Autodesk Fusion 360 part; units mm, degrees
(part 4 of 7)
  spline S1051 degree 3 poles (80.1455, 58.4684) (80.4873, 58.6658) (80.7712, 58.9498) (80.9687, 59.2916) knots 0 0 0 0 1 1 1 1
  spline S1052 degree 3 poles (81.2136, 60.9174) (81.1761, 61.0816) (81.1203, 61.241) (81.0472, 61.3928) knots 0 0 0 0 1 1 1 1
  spline S1053 degree 3 poles (81.2705, 60.4166) (81.2703, 60.5851) (81.2513, 60.7531) (81.2136, 60.9174) knots 0 0 0 0 1 1 1 1
  line L303 (70.73, 56.4437) -> (69.42, 56.4437)
  spline S1054 degree 3 poles (81.0472, 61.3928) (80.9743, 61.5446) (80.8845, 61.6878) (80.7795, 61.8196) knots 0 0 0 0 1 1 1 1
  spline S1055 degree 3 poles (80.7795, 61.8196) (80.6744, 61.9513) (80.5548, 62.0707) (80.423, 62.1757) knots 0 0 0 0 1 1 1 1
  spline S1056 degree 3 poles (79.9966, 62.4439) (79.8447, 62.517) (79.6851, 62.5728) (79.5207, 62.6103) knots 0 0 0 0 1 1 1 1
  line L304 (75.5752, 64.5037) -> (75.5752, 64.5037)
  spline S1057 degree 3 poles (68.6407, 56.8938) (68.8015, 56.6154) (69.0985, 56.4438) (69.42, 56.4437) knots 0 0 0 0 1 1 1 1
  spline S1058 degree 3 poles (71.5093, 57.7935) (71.3486, 58.072) (71.0515, 58.2436) (70.73, 58.2436) knots 0 0 0 0 1 1 1 1
  spline S1059 degree 3 poles (68.0149, 63.2438) (68.015, 62.6974) (68.2321, 62.1734) (68.6185, 61.7871) knots 0 0 0 0 1 1 1 1
  line L305 (79.0205, 62.6666) -> (79.0205, 62.6666)
  spline S1060 degree 3 poles (70.0753, 61.1835) (70.2552, 61.1836) (70.4343, 61.2072) (70.6081, 61.2538) knots 0 0 0 0 1 1 1 1
  spline S1061 degree 3 poles (71.1052, 61.4594) (71.261, 61.5496) (71.4043, 61.6597) (71.5315, 61.7871) knots 0 0 0 0 1 1 1 1
  spline S1062 degree 3 poles (71.1052, 65.0277) (70.9492, 65.1177) (70.7821, 65.1868) (70.6081, 65.2334) knots 0 0 0 0 1 1 1 1
  spline S1063 degree 3 poles (71.8592, 64.2737) (71.769, 64.4296) (71.6589, 64.5729) (71.5315, 64.7001) knots 0 0 0 0 1 1 1 1
  spline S1064 degree 3 poles (80.423, 62.1757) (80.2913, 62.2808) (80.1483, 62.3707) (79.9966, 62.4439) knots 0 0 0 0 1 1 1 1
  spline S1065 degree 3 poles (79.5207, 62.6103) (79.6851, 62.5728) (79.8447, 62.517) (79.9966, 62.4439) knots 0 0 0 0 1 1 1 1
  spline S1066 degree 3 poles (74.6843, 62.3524) (74.9206, 62.1162) (75.2411, 61.9834) (75.5752, 61.9834) knots 0 0 0 0 1 1 1 1
  spline S1067 degree 3 poles (77.0718, 59.2916) (77.2693, 58.9497) (77.5534, 58.6658) (77.8955, 58.4684) knots 0 0 0 0 1 1 1 1
  spline S1068 degree 3 poles (79.5207, 62.6103) (79.3566, 62.6477) (79.1888, 62.6666) (79.0205, 62.6666) knots 0 0 0 0 1 1 1 1
  line L306 (69.42, 56.4437) -> (70.73, 56.4437)
  line L307 (70.73, 58.2436) -> (69.42, 58.2436)
  spline S1069 degree 3 poles (68.6407, 57.7935) (68.8015, 58.072) (69.0985, 58.2436) (69.42, 58.2436) knots 0 0 0 0 1 1 1 1
  spline S1070 degree 3 poles (70.73, 58.2436) (71.0515, 58.2436) (71.3486, 58.072) (71.5093, 57.7935) knots 0 0 0 0 1 1 1 1
  spline S1071 degree 3 poles (70.0753, 65.3037) (69.5289, 65.3036) (69.0048, 65.0865) (68.6185, 64.7001) knots 0 0 0 0 1 1 1 1
  spline S1072 degree 3 poles (68.6185, 64.7001) (68.2322, 64.3139) (68.0151, 63.7901) (68.0149, 63.2438) knots 0 0 0 0 1 1 1 1
  spline S1073 degree 3 poles (70.6081, 61.2538) (70.7821, 61.3003) (70.9492, 61.3695) (71.1052, 61.4594) knots 0 0 0 0 1 1 1 1
  spline S1074 degree 3 poles (74.3148, 63.2438) (74.3148, 62.9094) (74.4477, 62.5887) (74.6843, 62.3524) knots 0 0 0 0 1 1 1 1
  spline S1075 degree 3 poles (76.7736, 63.633) (76.7326, 63.7588) (76.6721, 63.8774) (76.5943, 63.9844) knots 0 0 0 0 1 1 1 1
  line L308 (69.42, 58.2436) -> (70.73, 58.2436)
  spline S1076 degree 3 poles (72.0648, 63.7766) (72.0183, 63.9506) (71.9492, 64.1177) (71.8592, 64.2737) knots 0 0 0 0 1 1 1 1
  spline S1077 degree 3 poles (71.5315, 61.7871) (71.6589, 61.9143) (71.769, 62.0576) (71.8592, 62.2134) knots 0 0 0 0 1 1 1 1
  spline S1078 degree 3 poles (71.8592, 62.2134) (71.9492, 62.3694) (72.0183, 62.5365) (72.0648, 62.7105) knots 0 0 0 0 1 1 1 1
  line L309 (70.0753, 65.3037) -> (70.0753, 65.3037)
  spline S1079 degree 3 poles (76.8351, 63.2438) (76.8351, 63.376) (76.8144, 63.5073) (76.7736, 63.633) knots 0 0 0 0 1 1 1 1
  spline S1080 degree 3 poles (74.6843, 64.1347) (74.4479, 63.8985) (74.3149, 63.578) (74.3148, 63.2438) knots 0 0 0 0 1 1 1 1
  spline S1081 degree 3 poles (75.9643, 64.4417) (75.8387, 64.4826) (75.7074, 64.5036) (75.5752, 64.5037) knots 0 0 0 0 1 1 1 1
  spline S1082 degree 3 poles (70.73, 56.4437) (71.0515, 56.4438) (71.3486, 56.6154) (71.5093, 56.8938) knots 0 0 0 0 1 1 1 1
  spline S1083 degree 3 poles (68.6185, 61.7871) (69.0048, 61.4006) (69.5289, 61.1835) (70.0753, 61.1835) knots 0 0 0 0 1 1 1 1
  spline S1084 degree 3 poles (47.4048, 61.1856) (47.4049, 60.6391) (47.622, 60.1151) (48.0084, 59.7288) knots 0 0 0 0 1 1 1 1
  spline S1085 degree 3 poles (48.0084, 59.7288) (48.3946, 59.3425) (48.9184, 59.1254) (49.4647, 59.1252) knots 0 0 0 0 1 1 1 1
  spline S1086 degree 3 poles (46.1264, 56.7548) (45.9805, 56.4683) (45.6929, 56.2814) (45.3719, 56.2644) knots 0 0 0 0 1 1 1 1
  line L310 (49.1665, 54.3607) -> (50.4749, 54.4289)
  spline S1087 degree 3 poles (49.4647, 63.2454) (48.9185, 63.2454) (48.3947, 63.0284) (48.0084, 62.6423) knots 0 0 0 0 1 1 1 1
  spline S1088 degree 3 poles (49.4647, 59.1252) (49.6447, 59.1252) (49.824, 59.1489) (49.998, 59.1955) knots 0 0 0 0 1 1 1 1
  spline S1089 degree 3 poles (49.0724, 56.158) (48.752, 56.1404) (48.4651, 55.9536) (48.3195, 55.6676) knots 0 0 0 0 1 1 1 1
  spline S1090 degree 3 poles (51.2491, 60.1557) (51.339, 60.3115) (51.4081, 60.4785) (51.4547, 60.6523) knots 0 0 0 0 1 1 1 1
  line L311 (50.4749, 54.4289) -> (49.1665, 54.3607)
  spline S1091 degree 3 poles (51.4547, 60.6523) (51.5014, 60.8262) (51.525, 61.0055) (51.525, 61.1856) knots 0 0 0 0 1 1 1 1
  spline S1092 degree 3 poles (48.3665, 54.7699) (48.5411, 54.5006) (48.8459, 54.3447) (49.1665, 54.3607) knots 0 0 0 0 1 1 1 1
  spline S1093 degree 3 poles (79.9966, 62.4439) (80.1483, 62.3707) (80.2913, 62.2808) (80.423, 62.1757) knots 0 0 0 0 1 1 1 1
  spline S1094 degree 3 poles (50.4749, 54.4289) (50.7957, 54.4463) (51.0828, 54.6334) (51.2284, 54.9198) knots 0 0 0 0 1 1 1 1
  line L312 (50.3804, 56.2267) -> (50.3804, 56.2267)
  spline S1095 degree 3 poles (50.9214, 59.7288) (51.0488, 59.8561) (51.159, 59.9997) (51.2491, 60.1557) knots 0 0 0 0 1 1 1 1
  spline S1096 degree 3 poles (51.4547, 61.7189) (51.4081, 61.8927) (51.339, 62.0596) (51.2491, 62.2155) knots 0 0 0 0 1 1 1 1
  spline S1097 degree 3 poles (79.0205, 62.6666) (79.1888, 62.6666) (79.3566, 62.6477) (79.5207, 62.6103) knots 0 0 0 0 1 1 1 1
  spline S1098 degree 3 poles (50.9214, 62.6423) (50.7942, 62.7695) (50.6509, 62.8795) (50.4951, 62.9694) knots 0 0 0 0 1 1 1 1
  spline S1099 degree 3 poles (80.1455, 58.4684) (79.8035, 58.2708) (79.4155, 58.1667) (79.0205, 58.1666) knots 0 0 0 0 1 1 1 1
  spline S1100 degree 3 poles (46.0793, 57.6535) (46.2544, 57.3838) (46.2723, 57.0413) (46.1264, 56.7548) knots 0 0 0 0 1 1 1 1
  spline S1101 degree 3 poles (46.0793, 57.6535) (45.9042, 57.9232) (45.5985, 58.0791) (45.2773, 58.0622) knots 0 0 0 0 1 1 1 1
  spline S1102 degree 3 poles (54.0664, 62.3643) (53.8302, 62.128) (53.6975, 61.8075) (53.6975, 61.4734) knots 0 0 0 0 1 1 1 1
  spline S1103 degree 3 poles (51.2284, 54.9198) (51.0828, 54.6334) (50.7957, 54.4463) (50.4749, 54.4289) knots 0 0 0 0 1 1 1 1
  spline S1104 degree 3 poles (53.6975, 61.4734) (53.6975, 61.1393) (53.8302, 60.8188) (54.0664, 60.5825) knots 0 0 0 0 1 1 1 1
  line L313 (43.9694, 57.9935) -> (45.2773, 58.0622)
  spline S1105 degree 3 poles (49.998, 59.1955) (50.172, 59.2422) (50.3391, 59.3115) (50.4951, 59.4017) knots 0 0 0 0 1 1 1 1
  spline S1106 degree 3 poles (54.9574, 62.7333) (54.6232, 62.7333) (54.3027, 62.6006) (54.0664, 62.3643) knots 0 0 0 0 1 1 1 1
  spline S1107 degree 3 poles (51.2491, 62.2155) (51.159, 62.3715) (51.0488, 62.515) (50.9214, 62.6423) knots 0 0 0 0 1 1 1 1
  line L314 (50.3804, 56.2267) -> (49.0724, 56.158)
  spline S1108 degree 3 poles (50.4951, 62.9694) (50.3391, 63.0594) (50.172, 63.1286) (49.998, 63.1751) knots 0 0 0 0 1 1 1 1
  spline S1109 degree 3 poles (51.525, 61.1856) (51.525, 61.3656) (51.5014, 61.5449) (51.4547, 61.7189) knots 0 0 0 0 1 1 1 1
  spline S1110 degree 3 poles (54.9574, 60.2135) (55.2915, 60.2135) (55.612, 60.3462) (55.8483, 60.5825) knots 0 0 0 0 1 1 1 1
  spline S1111 degree 3 poles (80.423, 62.1757) (80.5548, 62.0707) (80.6744, 61.9513) (80.7795, 61.8196) knots 0 0 0 0 1 1 1 1
  line L315 (45.3719, 56.2644) -> (44.0634, 56.1957)
  spline S1112 degree 3 poles (80.9687, 59.2916) (80.7712, 58.9498) (80.4873, 58.6658) (80.1455, 58.4684) knots 0 0 0 0 1 1 1 1
  spline S1113 degree 3 poles (50.4951, 59.4017) (50.6509, 59.4916) (50.7942, 59.6016) (50.9214, 59.7288) knots 0 0 0 0 1 1 1 1
  spline S1114 degree 3 poles (51.1814, 55.8174) (51.0066, 56.087) (50.7013, 56.243) (50.3804, 56.2267) knots 0 0 0 0 1 1 1 1
  spline S1115 degree 3 poles (50.3804, 56.2267) (50.7013, 56.243) (51.0066, 56.087) (51.1814, 55.8174) knots 0 0 0 0 1 1 1 1
  spline S1116 degree 3 poles (49.998, 63.1751) (49.824, 63.2217) (49.6447, 63.2454) (49.4647, 63.2454) knots 0 0 0 0 1 1 1 1
  spline S1117 degree 3 poles (54.0664, 60.5825) (54.3027, 60.3462) (54.6232, 60.2135) (54.9574, 60.2135) knots 0 0 0 0 1 1 1 1
  spline S1118 degree 3 poles (56.2172, 61.4734) (56.2173, 61.6055) (56.1965, 61.7368) (56.1557, 61.8625) knots 0 0 0 0 1 1 1 1
  spline S1119 degree 3 poles (56.1557, 61.8625) (56.1149, 61.9883) (56.0546, 62.1069) (55.9769, 62.2139) knots 0 0 0 0 1 1 1 1
  spline S1120 degree 3 poles (48.3195, 55.6676) (48.174, 55.3814) (48.1919, 55.0393) (48.3665, 54.7699) knots 0 0 0 0 1 1 1 1
  spline S1121 degree 3 poles (48.3665, 54.7699) (48.1919, 55.0393) (48.174, 55.3814) (48.3195, 55.6676) knots 0 0 0 0 1 1 1 1
  spline S1122 degree 3 poles (55.8483, 60.5825) (56.0845, 60.8188) (56.2172, 61.1393) (56.2172, 61.4734) knots 0 0 0 0 1 1 1 1
  spline S1123 degree 3 poles (81.0472, 61.3928) (81.1203, 61.241) (81.1761, 61.0816) (81.2136, 60.9174) knots 0 0 0 0 1 1 1 1
  spline S1124 degree 3 poles (45.2773, 58.0622) (45.5985, 58.0791) (45.9042, 57.9232) (46.0793, 57.6535) knots 0 0 0 0 1 1 1 1
  spline S1125 degree 3 poles (44.0634, 56.1957) (43.7427, 56.1795) (43.4377, 56.3355) (43.263, 56.605) knots 0 0 0 0 1 1 1 1
  spline S1126 degree 3 poles (51.2284, 54.9198) (51.3739, 55.206) (51.356, 55.548) (51.1814, 55.8174) knots 0 0 0 0 1 1 1 1
  spline S1127 degree 3 poles (48.0084, 62.6423) (47.622, 62.256) (47.4049, 61.732) (47.4048, 61.1856) knots 0 0 0 0 1 1 1 1
  spline S1128 degree 3 poles (55.9769, 62.2139) (55.8991, 62.3208) (55.8049, 62.4148) (55.6979, 62.4925) knots 0 0 0 0 1 1 1 1
  spline S1129 degree 3 poles (81.2136, 60.9174) (81.2513, 60.7531) (81.2703, 60.5851) (81.2705, 60.4166) knots 0 0 0 0 1 1 1 1
  spline S1130 degree 3 poles (48.3195, 55.6676) (48.4651, 55.9536) (48.752, 56.1404) (49.0724, 56.158) knots 0 0 0 0 1 1 1 1
  line L316 (49.4647, 63.2454) -> (49.4647, 63.2454)
  spline S1131 degree 3 poles (55.6979, 62.4925) (55.5909, 62.5703) (55.4723, 62.6308) (55.3465, 62.6718) knots 0 0 0 0 1 1 1 1
  spline S1132 degree 3 poles (83.1639, 74.4375) (82.8425, 74.4431) (82.5425, 74.2768) (82.3769, 74.0013) knots 0 0 0 0 1 1 1 1
  spline S1133 degree 3 poles (81.2705, 60.4166) (81.2704, 60.0216) (81.1663, 59.6336) (80.9687, 59.2916) knots 0 0 0 0 1 1 1 1
  spline S1134 degree 3 poles (49.1665, 54.3607) (48.8459, 54.3447) (48.5411, 54.5006) (48.3665, 54.7699) knots 0 0 0 0 1 1 1 1
  spline S1135 degree 3 poles (80.7795, 61.8196) (80.8845, 61.6878) (80.9743, 61.5446) (81.0472, 61.3928) knots 0 0 0 0 1 1 1 1
  spline S1136 degree 3 poles (51.1814, 55.8174) (51.356, 55.548) (51.3739, 55.206) (51.2284, 54.9198) knots 0 0 0 0 1 1 1 1
  line L317 (45.2773, 58.0622) -> (45.2773, 58.0622)
  spline S1137 degree 3 poles (43.216, 57.5031) (43.3616, 57.7893) (43.6487, 57.9762) (43.9694, 57.9935) knots 0 0 0 0 1 1 1 1
  spline S1138 degree 3 poles (43.263, 56.605) (43.0881, 56.8745) (43.0702, 57.2168) (43.216, 57.5031) knots 0 0 0 0 1 1 1 1
  line L318 (49.0724, 56.158) -> (50.3804, 56.2267)
  line L319 (64.4203, 60.3438) -> (65.7303, 60.3438)
  spline S1139 degree 3 poles (65.7303, 60.3438) (66.0518, 60.3437) (66.3489, 60.1721) (66.5096, 59.8937) knots 0 0 0 0 1 1 1 1
  spline S1140 degree 3 poles (66.5096, 58.9934) (66.6705, 59.272) (66.6705, 59.6151) (66.5096, 59.8937) knots 0 0 0 0 1 1 1 1
  line L320 (64.4203, 58.5439) -> (65.7303, 58.5439)
  spline S1141 degree 3 poles (65.4663, 62.3524) (65.7026, 62.5888) (65.8354, 62.9095) (65.8352, 63.2438) knots 0 0 0 0 1 1 1 1
  spline S1142 degree 3 poles (64.4203, 58.5439) (64.0987, 58.5436) (63.8015, 58.715) (63.6405, 58.9934) knots 0 0 0 0 1 1 1 1
  spline S1143 degree 3 poles (65.8352, 63.2438) (65.8351, 63.376) (65.8142, 63.5073) (65.7732, 63.633) knots 0 0 0 0 1 1 1 1
  spline S1144 degree 3 poles (43.1705, 60.4166) (43.1703, 60.2725) (43.1563, 60.1287) (43.1286, 59.9872) knots 0 0 0 0 1 1 1 1
  line L321 (67.0651, 54.4439) -> (67.0651, 54.9234)
  spline S1145 degree 3 poles (64.5748, 64.5037) (64.2407, 64.5037) (63.9202, 64.371) (63.6839, 64.1347) knots 0 0 0 0 1 1 1 1
  line L322 (70.0851, 48.9434) -> (68.4852, 48.9434)
  spline S1146 degree 3 poles (85.2273, 73.052) (85.3924, 73.3274) (85.3983, 73.6698) (85.2428, 73.9507) knots 0 0 0 0 1 1 1 1
  spline S1147 degree 3 poles (85.2428, 73.9507) (85.0874, 74.2315) (84.7943, 74.4083) (84.4734, 74.4147) knots 0 0 0 0 1 1 1 1
  spline S1148 degree 3 poles (65.7732, 63.633) (65.7324, 63.7587) (65.6721, 63.8773) (65.5944, 63.9844) knots 0 0 0 0 1 1 1 1
  spline S1149 degree 3 poles (63.6405, 58.9934) (63.4797, 59.272) (63.4797, 59.6151) (63.6405, 59.8937) knots 0 0 0 0 1 1 1 1
  line L323 (68.4852, 48.9434) -> (67.5349, 49.8436)
  spline S1150 degree 3 poles (112.8644, 55.9265) (112.9902, 55.8855) (113.1088, 55.825) (113.2158, 55.7471) knots 0 0 0 0 1 1 1 1
  line L324 (65.7303, 58.5439) -> (64.4203, 58.5439)
  spline S1151 degree 3 poles (43.1136, 60.9174) (43.1513, 60.7531) (43.1703, 60.5851) (43.1705, 60.4166) knots 0 0 0 0 1 1 1 1
  spline S1152 degree 3 poles (63.6405, 58.9934) (63.8015, 58.715) (64.0987, 58.5436) (64.4203, 58.5439) knots 0 0 0 0 1 1 1 1
  spline S1153 degree 3 poles (63.6405, 59.8937) (63.4797, 59.6151) (63.4797, 59.272) (63.6405, 58.9934) knots 0 0 0 0 1 1 1 1
  spline S1154 degree 3 poles (64.5748, 61.9834) (64.9092, 61.9833) (65.2298, 62.116) (65.4663, 62.3524) knots 0 0 0 0 1 1 1 1
  spline S1155 degree 3 poles (65.3159, 64.2629) (65.2089, 64.3406) (65.0903, 64.4009) (64.9645, 64.4417) knots 0 0 0 0 1 1 1 1
  spline S1156 degree 3 poles (55.3465, 62.6718) (55.2208, 62.7126) (55.0895, 62.7333) (54.9574, 62.7333) knots 0 0 0 0 1 1 1 1
  line L325 (45.2773, 58.0622) -> (43.9694, 57.9935)
  spline S1157 degree 3 poles (43.9694, 57.9935) (43.6487, 57.9762) (43.3616, 57.7893) (43.216, 57.5031) knots 0 0 0 0 1 1 1 1
  line L326 (44.0634, 56.1957) -> (45.3719, 56.2644)
  spline S1158 degree 3 poles (113.2158, 55.7471) (113.3227, 55.6695) (113.4167, 55.5755) (113.4943, 55.4686) knots 0 0 0 0 1 1 1 1
  spline S1159 degree 3 poles (84.4418, 72.6148) (84.7629, 72.61) (85.0622, 72.7766) (85.2273, 73.052) knots 0 0 0 0 1 1 1 1
  spline S1160 degree 3 poles (113.4943, 55.4686) (113.572, 55.3616) (113.6323, 55.243) (113.6731, 55.1172) knots 0 0 0 0 1 1 1 1
  spline S1161 degree 3 poles (64.9645, 64.4417) (64.8387, 64.4827) (64.7072, 64.5036) (64.5748, 64.5037) knots 0 0 0 0 1 1 1 1
  spline S1162 degree 3 poles (65.5944, 63.9844) (65.5168, 64.0912) (65.4228, 64.1852) (65.3159, 64.2629) knots 0 0 0 0 1 1 1 1
  line L327 (67.5349, 49.8436) -> (64.5051, 49.8436)
  spline S1163 degree 3 poles (65.7303, 58.5439) (66.0517, 58.5438) (66.3488, 58.7152) (66.5096, 58.9934) knots 0 0 0 0 1 1 1 1
  spline S1164 degree 3 poles (66.5096, 58.9934) (66.3488, 58.7152) (66.0517, 58.5438) (65.7303, 58.5439) knots 0 0 0 0 1 1 1 1
  line L328 (84.4734, 74.4147) -> (83.1639, 74.4375)
  line L329 (54.9574, 62.7333) -> (54.9574, 62.7333)
  spline S1165 degree 3 poles (63.315, 63.2438) (63.3148, 62.9095) (63.4476, 62.5888) (63.6839, 62.3524) knots 0 0 0 0 1 1 1 1
  line L330 (64.5748, 64.5037) -> (64.5748, 64.5037)
  line L331 (67.0651, 54.9234) -> (67.585, 55.4438)
  spline S1166 degree 3 poles (82.3769, 74.0013) (82.2112, 73.7258) (82.2051, 73.3829) (82.3608, 73.1016) knots 0 0 0 0 1 1 1 1
  line L332 (64.4203, 60.3438) -> (64.4203, 60.3438)
  spline S1167 degree 3 poles (45.3719, 56.2644) (45.6929, 56.2814) (45.9805, 56.4683) (46.1264, 56.7548) knots 0 0 0 0 1 1 1 1
  spline S1168 degree 3 poles (113.7351, 54.7281) (113.7351, 54.3939) (113.6024, 54.0735) (113.3662, 53.8372) knots 0 0 0 0 1 1 1 1
  spline S1169 degree 3 poles (113.6731, 55.1172) (113.7141, 54.9915) (113.735, 54.8602) (113.7351, 54.7281) knots 0 0 0 0 1 1 1 1
  spline S1170 degree 3 poles (66.5096, 59.8937) (66.3489, 60.1721) (66.0518, 60.3437) (65.7303, 60.3438) knots 0 0 0 0 1 1 1 1
  spline S1171 degree 3 poles (64.4203, 60.3438) (64.0986, 60.3439) (63.8013, 60.1723) (63.6405, 59.8937) knots 0 0 0 0 1 1 1 1
  spline S1172 degree 3 poles (43.263, 56.605) (43.4377, 56.3355) (43.7427, 56.1795) (44.0634, 56.1957) knots 0 0 0 0 1 1 1 1
  line L333 (64.5051, 49.8436) -> (64.5051, 54.4439)
  spline S1173 degree 3 poles (112.4748, 55.9879) (112.6071, 55.988) (112.7385, 55.9673) (112.8644, 55.9265) knots 0 0 0 0 1 1 1 1
  line L334 (65.7303, 60.3438) -> (64.4203, 60.3438)
  spline S1174 degree 3 poles (71.0783, 48.6106) (70.8006, 48.842) (70.4462, 48.9607) (70.0851, 48.9434) knots 0 0 0 0 1 1 1 1
  spline S1175 degree 3 poles (82.3608, 73.1016) (82.5167, 72.8204) (82.8108, 72.6437) (83.1324, 72.6381) knots 0 0 0 0 1 1 1 1
  spline S1176 degree 3 poles (112.4748, 53.4677) (112.1405, 53.4678) (111.8201, 53.6007) (111.5839, 53.8372) knots 0 0 0 0 1 1 1 1
  line L335 (83.1324, 72.6381) -> (84.4418, 72.6148)
  spline S1177 degree 3 poles (63.6405, 59.8937) (63.8013, 60.1723) (64.0986, 60.3439) (64.4203, 60.3438) knots 0 0 0 0 1 1 1 1
  spline S1178 degree 3 poles (43.216, 57.5031) (43.0702, 57.2168) (43.0881, 56.8745) (43.263, 56.605) knots 0 0 0 0 1 1 1 1
  spline S1179 degree 3 poles (46.1264, 56.7548) (46.2723, 57.0413) (46.2544, 57.3838) (46.0793, 57.6535) knots 0 0 0 0 1 1 1 1
  spline S1180 degree 3 poles (113.3662, 53.8372) (113.1298, 53.6006) (112.8091, 53.4677) (112.4748, 53.4677) knots 0 0 0 0 1 1 1 1
  spline S1181 degree 3 poles (66.5096, 59.8937) (66.6705, 59.6151) (66.6705, 59.272) (66.5096, 58.9934) knots 0 0 0 0 1 1 1 1
  spline S1182 degree 3 poles (63.6839, 62.3524) (63.9202, 62.1162) (64.2407, 61.9834) (64.5748, 61.9834) knots 0 0 0 0 1 1 1 1
  line L336 (43.1286, 59.9872) -> (43.1286, 59.9872)
  line L337 (64.5051, 54.4439) -> (67.0651, 54.4439)
  spline S1183 degree 3 poles (63.6839, 64.1347) (63.4477, 63.8984) (63.315, 63.578) (63.315, 63.2438) knots 0 0 0 0 1 1 1 1
  line L338 (40.7288, 58.8255) -> (40.783, 58.2033)
  spline S1184 degree 3 poles (101.4816, 56.3719) (101.6139, 56.372) (101.7454, 56.3512) (101.8713, 56.3104) knots 0 0 0 0 1 1 1 1
  spline S1185 degree 3 poles (40.9205, 58.1666) (41.3155, 58.1667) (41.7035, 58.2708) (42.0455, 58.4684) knots 0 0 0 0 1 1 1 1
  spline S1186 degree 3 poles (102.68, 55.5012) (102.7208, 55.3755) (102.7415, 55.2442) (102.7415, 55.112) knots 0 0 0 0 1 1 1 1
  line L339 (112.4748, 55.9879) -> (112.4748, 55.9879)
  spline S1187 degree 3 poles (109.0383, 54.9198) (109.0383, 54.7397) (109.0146, 54.5604) (108.968, 54.3865) knots 0 0 0 0 1 1 1 1
  line L340 (106.9784, 56.9801) -> (106.9784, 56.9801)
  spline S1188 degree 3 poles (111.2149, 54.7281) (111.2149, 55.0622) (111.3476, 55.3827) (111.5839, 55.619) knots 0 0 0 0 1 1 1 1
  spline S1189 degree 3 poles (111.5839, 55.619) (111.8201, 55.8552) (112.1406, 55.988) (112.4748, 55.9879) knots 0 0 0 0 1 1 1 1
  spline S1190 degree 3 poles (38.6705, 60.4166) (38.6704, 60.0217) (38.7743, 59.6337) (38.9718, 59.2916) knots 0 0 0 0 1 1 1 1
  spline S1191 degree 3 poles (106.9784, 52.86) (106.4321, 52.8599) (105.9081, 53.0768) (105.5217, 53.463) knots 0 0 0 0 1 1 1 1
  spline S1192 degree 3 poles (40.9205, 62.6666) (40.5255, 62.6667) (40.1375, 62.5628) (39.7955, 62.3653) knots 0 0 0 0 1 1 1 1
  spline S1193 degree 3 poles (108.0084, 56.7037) (108.1643, 56.6137) (108.3078, 56.5038) (108.4352, 56.3766) knots 0 0 0 0 1 1 1 1
  spline S1194 degree 3 poles (105.5217, 53.463) (105.1353, 53.8494) (104.9181, 54.3734) (104.9181, 54.9198) knots 0 0 0 0 1 1 1 1
  spline S1195 degree 3 poles (42.0455, 58.4684) (42.3874, 58.6658) (42.6713, 58.9498) (42.8687, 59.2916) knots 0 0 0 0 1 1 1 1
  spline S1196 degree 3 poles (43.1705, 60.4166) (43.1703, 60.5851) (43.1513, 60.7531) (43.1136, 60.9174) knots 0 0 0 0 1 1 1 1
  spline S1197 degree 3 poles (42.9472, 61.3928) (42.8743, 61.5446) (42.7845, 61.6878) (42.6795, 61.8196) knots 0 0 0 0 1 1 1 1
  spline S1198 degree 3 poles (42.323, 62.1757) (42.1914, 62.2808) (42.0484, 62.3707) (41.8967, 62.4439) knots 0 0 0 0 1 1 1 1
  spline S1199 degree 3 poles (106.9784, 56.9801) (107.1585, 56.9801) (107.3378, 56.9565) (107.5118, 56.9099) knots 0 0 0 0 1 1 1 1
  spline S1200 degree 3 poles (38.9718, 61.5416) (38.7743, 61.1996) (38.6704, 60.8116) (38.6705, 60.4166) knots 0 0 0 0 1 1 1 1
  line L341 (106.149, 49.9459) -> (107.4585, 49.8999)
  spline S1201 degree 3 poles (41.4207, 62.6103) (41.2566, 62.6477) (41.0888, 62.6666) (40.9205, 62.6666) knots 0 0 0 0 1 1 1 1
  line L342 (40.9205, 62.6666) -> (40.9205, 62.6666)
  spline S1202 degree 3 poles (102.7415, 55.112) (102.7415, 54.7779) (102.6088, 54.4574) (102.3725, 54.2211) knots 0 0 0 0 1 1 1 1
  spline S1203 degree 3 poles (108.2218, 49.423) (108.3726, 49.1391) (108.3606, 48.7964) (108.1903, 48.5238) knots 0 0 0 0 1 1 1 1
  spline S1204 degree 3 poles (104.9181, 54.9198) (104.9181, 55.4662) (105.1353, 55.9902) (105.5217, 56.3766) knots 0 0 0 0 1 1 1 1
  spline S1205 degree 3 poles (108.4352, 56.3766) (108.5624, 56.2492) (108.6724, 56.1057) (108.7623, 55.9497) knots 0 0 0 0 1 1 1 1
  spline S1206 degree 3 poles (107.4585, 49.8999) (107.7799, 49.8887) (108.0708, 49.7069) (108.2218, 49.423) knots 0 0 0 0 1 1 1 1
  spline S1207 degree 3 poles (105.3233, 48.6241) (105.1724, 48.9079) (105.1845, 49.2506) (105.3548, 49.5232) knots 0 0 0 0 1 1 1 1
  spline S1208 degree 3 poles (107.5118, 56.9099) (107.6856, 56.8631) (107.8525, 56.7938) (108.0084, 56.7037) knots 0 0 0 0 1 1 1 1
  spline S1209 degree 3 poles (100.5907, 56.0029) (100.827, 56.2392) (101.1475, 56.3719) (101.4816, 56.3719) knots 0 0 0 0 1 1 1 1
  spline S1210 degree 3 poles (108.7623, 53.8899) (108.6724, 53.7339) (108.5624, 53.5904) (108.4352, 53.463) knots 0 0 0 0 1 1 1 1
  spline S1211 degree 3 poles (108.0084, 53.1359) (107.8525, 53.046) (107.6856, 52.9768) (107.5118, 52.9303) knots 0 0 0 0 1 1 1 1
  line L343 (39.5418, 58.7216) -> (40.7288, 58.8255)
  spline S1212 degree 3 poles (108.1903, 48.5238) (108.0199, 48.251) (107.7169, 48.0899) (107.3955, 48.1011) knots 0 0 0 0 1 1 1 1
  line L344 (107.3955, 48.1011) -> (106.0865, 48.1471)
  spline S1213 degree 3 poles (102.3725, 54.2211) (102.1363, 53.9847) (101.8158, 53.8518) (101.4816, 53.8516) knots 0 0 0 0 1 1 1 1
  spline S1214 degree 3 poles (106.0865, 48.1471) (105.7652, 48.1583) (105.4742, 48.3401) (105.3233, 48.6241) knots 0 0 0 0 1 1 1 1
  spline S1215 degree 3 poles (105.3548, 49.5232) (105.525, 49.7959) (105.8278, 49.957) (106.149, 49.9459) knots 0 0 0 0 1 1 1 1
  spline S1216 degree 3 poles (42.6795, 61.8196) (42.5744, 61.9513) (42.4548, 62.0707) (42.323, 62.1757) knots 0 0 0 0 1 1 1 1
  line L345 (106.149, 49.9459) -> (106.149, 49.9459)
  spline S1217 degree 3 poles (107.5118, 52.9303) (107.3378, 52.8836) (107.1585, 52.86) (106.9784, 52.86) knots 0 0 0 0 1 1 1 1
  spline S1218 degree 3 poles (42.8687, 59.2916) (43.0663, 59.6336) (43.1704, 60.0216) (43.1705, 60.4166) knots 0 0 0 0 1 1 1 1
  spline S1219 degree 3 poles (41.8967, 62.4439) (41.7447, 62.517) (41.5851, 62.5728) (41.4207, 62.6103) knots 0 0 0 0 1 1 1 1
  spline S1220 degree 3 poles (102.2222, 56.1311) (102.3292, 56.0535) (102.4234, 55.9595) (102.5012, 55.8526) knots 0 0 0 0 1 1 1 1
  spline S1221 degree 3 poles (43.1136, 60.9174) (43.0761, 61.0816) (43.0203, 61.241) (42.9472, 61.3928) knots 0 0 0 0 1 1 1 1
  spline S1222 degree 3 poles (43.1286, 59.9872) (43.3562, 59.7691) (43.6573, 59.6443) (43.9725, 59.6373) knots 0 0 0 0 1 1 1 1
  spline S1223 degree 3 poles (101.8713, 56.3104) (101.9969, 56.2694) (102.1153, 56.2089) (102.2222, 56.1311) knots 0 0 0 0 1 1 1 1
  spline S1224 degree 3 poles (101.4816, 53.8516) (101.1474, 53.8518) (100.8269, 53.9847) (100.5907, 54.2211) knots 0 0 0 0 1 1 1 1
  spline S1225 degree 3 poles (105.5217, 56.3766) (105.908, 56.763) (106.432, 56.9801) (106.9784, 56.9801) knots 0 0 0 0 1 1 1 1
  spline S1226 degree 3 poles (45.2324, 60.8977) (45.2324, 61.2319) (45.0997, 61.5523) (44.8634, 61.7886) knots 0 0 0 0 1 1 1 1
  spline S1227 degree 3 poles (44.8634, 60.0068) (45.0997, 60.2431) (45.2324, 60.5636) (45.2324, 60.8977) knots 0 0 0 0 1 1 1 1
  spline S1228 degree 3 poles (111.5839, 53.8372) (111.3476, 54.0735) (111.2149, 54.3939) (111.2149, 54.7281) knots 0 0 0 0 1 1 1 1
  spline S1229 degree 3 poles (102.5012, 55.8526) (102.5789, 55.7455) (102.6392, 55.6269) (102.68, 55.5012) knots 0 0 0 0 1 1 1 1
  line L346 (101.4816, 56.3719) -> (101.4816, 56.3719)
  spline S1230 degree 3 poles (108.7623, 55.9497) (108.8523, 55.7939) (108.9214, 55.6269) (108.968, 55.4531) knots 0 0 0 0 1 1 1 1
  spline S1231 degree 3 poles (108.968, 54.3865) (108.9214, 54.2127) (108.8523, 54.0457) (108.7623, 53.8899) knots 0 0 0 0 1 1 1 1
  spline S1232 degree 3 poles (108.4352, 53.463) (108.3078, 53.3358) (108.1643, 53.2258) (108.0084, 53.1359) knots 0 0 0 0 1 1 1 1
  spline S1233 degree 3 poles (40.783, 58.2033) (40.8284, 58.1896) (40.8743, 58.1774) (40.9205, 58.1666) knots 0 0 0 0 1 1 1 1
  spline S1234 degree 3 poles (108.968, 55.4531) (109.0146, 55.2792) (109.0383, 55.0999) (109.0383, 54.9198) knots 0 0 0 0 1 1 1 1
  spline S1235 degree 3 poles (100.2218, 55.112) (100.2218, 55.4462) (100.3545, 55.7666) (100.5907, 56.0029) knots 0 0 0 0 1 1 1 1
  spline S1236 degree 3 poles (38.9718, 59.2916) (39.1259, 59.0689) (39.319, 58.8758) (39.5418, 58.7216) knots 0 0 0 0 1 1 1 1
  spline S1237 degree 3 poles (100.5907, 54.2211) (100.3545, 54.4574) (100.2218, 54.7779) (100.2218, 55.112) knots 0 0 0 0 1 1 1 1
  spline S1238 degree 3 poles (39.7955, 62.3653) (39.4534, 62.1678) (39.1693, 61.8837) (38.9718, 61.5416) knots 0 0 0 0 1 1 1 1
  spline S1239 degree 3 poles (42.9307, 61.4248) (42.9363, 61.4142) (42.9418, 61.4035) (42.9472, 61.3928) knots 0 0 0 0 1 1 1 1
  spline S1240 degree 3 poles (37.0814, 51.4642) (37.3177, 51.7005) (37.4504, 52.021) (37.4504, 52.3551) knots 0 0 0 0 1 1 1 1
  line L347 (101.2258, 52.2192) -> (102.5348, 52.1732)
  line L348 (85.9461, 52.4858) -> (90.9453, 52.3985)
  spline S1241 degree 3 poles (100.431, 51.7965) (100.6014, 52.0693) (100.9044, 52.2304) (101.2258, 52.2192) knots 0 0 0 0 1 1 1 1
  line L349 (96.4096, 50.3025) -> (96.3894, 49.1527)
  line L350 (98.964, 49.1077) -> (98.8839, 44.5085)
  line L351 (96.3093, 44.5535) -> (96.2928, 43.6037)
  spline S1242 degree 3 poles (71.5315, 47.7001) (71.5499, 47.6772) (71.5679, 47.654) (71.5853, 47.6303) knots 0 0 0 0 1 1 1 1
  spline S1243 degree 3 poles (71.1052, 44.4595) (70.9492, 44.3695) (70.7821, 44.3003) (70.6081, 44.2538) knots 0 0 0 0 1 1 1 1
  line L352 (90.9453, 52.3985) -> (91.4363, 51.8895)
  line L353 (98.8839, 44.5085) -> (96.3093, 44.5535)
  line L354 (96.2928, 43.6037) -> (94.9265, 43.6275)
  spline S1244 degree 3 poles (37.4504, 52.3551) (37.4505, 52.4874) (37.4297, 52.6189) (37.3889, 52.7447) knots 0 0 0 0 1 1 1 1
  spline S1245 degree 3 poles (32.4957, 50.8461) (32.5856, 51.002) (32.6548, 51.1689) (32.7014, 51.3428) knots 0 0 0 0 1 1 1 1
  line L355 (91.9101, 50.3811) -> (96.4096, 50.3025)
  spline S1246 degree 3 poles (94.9265, 43.6275) (94.943, 43.5979) (94.9584, 43.5678) (94.9725, 43.537) knots 0 0 0 0 1 1 1 1
  spline S1247 degree 3 poles (91.5577, 50.5325) (91.65, 50.4367) (91.7771, 50.3821) (91.9101, 50.3811) knots 0 0 0 0 1 1 1 1
  spline S1248 degree 3 poles (44.8634, 61.7886) (44.6271, 62.0249) (44.3066, 62.1576) (43.9725, 62.1576) knots 0 0 0 0 1 1 1 1
  spline S1249 degree 3 poles (95.0345, 43.1474) (95.0343, 42.8132) (94.9014, 42.4927) (94.665, 42.2565) knots 0 0 0 0 1 1 1 1
  line L356 (32.6445, 52.5468) -> (32.1722, 52.5055)
  spline S1250 degree 3 poles (103.2665, 50.7971) (103.0962, 50.5243) (102.7932, 50.3631) (102.4717, 50.3743) knots 0 0 0 0 1 1 1 1
  spline S1251 degree 3 poles (71.1052, 48.0277) (71.261, 47.9376) (71.4043, 47.8274) (71.5315, 47.7001) knots 0 0 0 0 1 1 1 1
  spline S1252 degree 3 poles (94.665, 42.2565) (94.4287, 42.0202) (94.1082, 41.8875) (93.7741, 41.8875) knots 0 0 0 0 1 1 1 1
  spline S1253 degree 3 poles (101.1628, 50.4203) (100.8415, 50.4315) (100.5506, 50.6131) (100.3995, 50.8968) knots 0 0 0 0 1 1 1 1
  spline S1254 degree 3 poles (93.7741, 41.8875) (93.4399, 41.8875) (93.1195, 42.0202) (92.8832, 42.2565) knots 0 0 0 0 1 1 1 1
  spline S1255 degree 3 poles (92.8832, 42.2565) (92.6469, 42.4928) (92.5142, 42.8132) (92.5142, 43.1474) knots 0 0 0 0 1 1 1 1
  spline S1256 degree 3 poles (43.9725, 59.6373) (44.3067, 59.6375) (44.6272, 59.7704) (44.8634, 60.0068) knots 0 0 0 0 1 1 1 1
  line L357 (102.4717, 50.3743) -> (101.1628, 50.4203)
  spline S1257 degree 3 poles (92.5142, 43.1474) (92.5458, 43.3343) (92.6191, 43.5116) (92.7287, 43.6662) knots 0 0 0 0 1 1 1 1
  spline S1258 degree 3 poles (90.2735, 43.7091) (90.3117, 43.5568) (90.3323, 43.4005) (90.335, 43.2435) knots 0 0 0 0 1 1 1 1
  spline S1259 degree 3 poles (91.4192, 50.8901) (91.4154, 50.7571) (91.4653, 50.6282) (91.5577, 50.5325) knots 0 0 0 0 1 1 1 1
  spline S1260 degree 3 poles (70.6081, 44.2538) (70.4343, 44.2072) (70.2552, 44.1836) (70.0753, 44.1835) knots 0 0 0 0 1 1 1 1
  line L358 (101.2258, 52.2192) -> (101.2258, 52.2192)
  spline S1261 degree 3 poles (70.0753, 44.1835) (69.5289, 44.1835) (69.0048, 44.4006) (68.6185, 44.7871) knots 0 0 0 0 1 1 1 1
  line L359 (91.4363, 51.8895) -> (91.4192, 50.8901)
  spline S1262 degree 3 poles (68.6185, 47.7001) (69.0048, 48.0865) (69.5289, 48.3036) (70.0753, 48.3037) knots 0 0 0 0 1 1 1 1
  spline S1263 degree 3 poles (71.5315, 44.7871) (71.4043, 44.6597) (71.261, 44.5496) (71.1052, 44.4595) knots 0 0 0 0 1 1 1 1
  spline S1264 degree 3 poles (43.0816, 61.7886) (43.0125, 61.676) (42.9616, 61.5532) (42.9307, 61.4248) knots 0 0 0 0 1 1 1 1
  spline S1265 degree 3 poles (68.0149, 46.2438) (68.0151, 46.7901) (68.2322, 47.3139) (68.6185, 47.7001) knots 0 0 0 0 1 1 1 1
  spline S1266 degree 3 poles (103.2981, 51.6962) (103.4489, 51.4124) (103.4368, 51.0696) (103.2665, 50.7971) knots 0 0 0 0 1 1 1 1
  line L360 (32.1722, 52.5055) -> (32.0952, 53.3886)
  line L361 (37.283, 52.953) -> (35.0991, 52.7618)
  line L362 (96.3894, 49.1527) -> (98.964, 49.1077)
  spline S1267 degree 3 poles (32.7014, 51.3428) (32.748, 51.5167) (32.7716, 51.696) (32.7716, 51.8761) knots 0 0 0 0 1 1 1 1
  spline S1268 degree 3 poles (34.9307, 52.3551) (34.9307, 52.021) (35.0634, 51.7005) (35.2996, 51.4642) knots 0 0 0 0 1 1 1 1
  spline S1269 degree 3 poles (68.6185, 44.7871) (68.2321, 45.1734) (68.015, 45.6974) (68.0149, 46.2438) knots 0 0 0 0 1 1 1 1
  spline S1270 degree 3 poles (35.2996, 51.4642) (35.5359, 51.2279) (35.8564, 51.0952) (36.1905, 51.0952) knots 0 0 0 0 1 1 1 1
  spline S1271 degree 3 poles (36.1905, 51.0952) (36.5247, 51.0952) (36.8451, 51.2279) (37.0814, 51.4642) knots 0 0 0 0 1 1 1 1
  spline S1272 degree 3 poles (100.3995, 50.8968) (100.2485, 51.1808) (100.2605, 51.5238) (100.431, 51.7965) knots 0 0 0 0 1 1 1 1
  spline S1273 degree 3 poles (94.9725, 43.537) (95.0135, 43.4112) (95.0344, 43.2797) (95.0345, 43.1474) knots 0 0 0 0 1 1 1 1
  spline S1274 degree 3 poles (43.9725, 62.1576) (43.6384, 62.1576) (43.3179, 62.0249) (43.0816, 61.7886) knots 0 0 0 0 1 1 1 1
  line L363 (92.7287, 43.6662) -> (90.2735, 43.7091)
  spline S1275 degree 3 poles (90.335, 43.2435) (90.335, 43.0634) (90.3114, 42.8841) (90.2647, 42.7102) knots 0 0 0 0 1 1 1 1
  spline S1276 degree 3 poles (102.5348, 52.1732) (102.8562, 52.162) (103.1471, 51.9801) (103.2981, 51.6962) knots 0 0 0 0 1 1 1 1
  line L364 (71.5853, 47.6303) -> (71.5853, 47.6934)
  spline S1277 degree 3 poles (70.0753, 48.3037) (70.2552, 48.3036) (70.4343, 48.28) (70.6081, 48.2334) knots 0 0 0 0 1 1 1 1
  spline S1278 degree 3 poles (42.9472, 61.3928) (43.0203, 61.241) (43.0761, 61.0816) (43.1136, 60.9174) knots 0 0 0 0 1 1 1 1
  spline S1279 degree 3 poles (70.6081, 48.2334) (70.7821, 48.1869) (70.9492, 48.1177) (71.1052, 48.0277) knots 0 0 0 0 1 1 1 1
  spline S1280 degree 3 poles (71.5853, 47.6934) (71.5371, 48.0518) (71.3562, 48.3792) (71.0783, 48.6106) knots 0 0 0 0 1 1 1 1
  spline S1281 degree 3 poles (32.7014, 52.4088) (32.6841, 52.4555) (32.6651, 52.5015) (32.6445, 52.5468) knots 0 0 0 0 1 1 1 1
  spline S1282 degree 3 poles (37.3889, 52.7447) (37.3601, 52.8173) (37.3247, 52.887) (37.283, 52.953) knots 0 0 0 0 1 1 1 1
  spline S1283 degree 3 poles (35.0991, 52.7618) (35.0196, 52.6372) (34.9625, 52.4995) (34.9307, 52.3551) knots 0 0 0 0 1 1 1 1
  spline S1284 degree 3 poles (32.7716, 51.8761) (32.7716, 52.056) (32.7479, 52.2351) (32.7014, 52.4088) knots 0 0 0 0 1 1 1 1
  spline S1285 degree 3 poles (89.732, 41.7868) (89.6046, 41.6595) (89.4611, 41.5496) (89.3051, 41.4596) knots 0 0 0 0 1 1 1 1
  spline S1286 degree 3 poles (88.808, 45.2336) (88.982, 45.1869) (89.1491, 45.1176) (89.3051, 45.0274) knots 0 0 0 0 1 1 1 1
  spline S1287 degree 3 poles (76.7736, 46.633) (76.8144, 46.5073) (76.8351, 46.376) (76.8351, 46.2438) knots 0 0 0 0 1 1 1 1
  line L365 (88.332, 45.9431) -> (86.7327, 45.971)
  spline S1288 degree 3 poles (26.2516, 50.656) (26.174, 50.5489) (26.08, 50.4547) (25.9731, 50.3769) knots 0 0 0 0 1 1 1 1
  line L366 (78.0851, 52.2936) -> (80.6602, 52.2936)
  spline S1289 degree 3 poles (89.3196, 45.5927) (89.0459, 45.8291) (88.6935, 45.9541) (88.332, 45.9431) knots 0 0 0 0 1 1 1 1
  spline S1290 degree 3 poles (25.6217, 50.1981) (25.496, 50.1573) (25.3647, 50.1366) (25.2326, 50.1366) knots 0 0 0 0 1 1 1 1
  spline S1291 degree 3 poles (76.7173, 46.7436) (76.7378, 46.7076) (76.7566, 46.6707) (76.7736, 46.633) knots 0 0 0 0 1 1 1 1
  spline S1292 degree 3 poles (26.4309, 51.0074) (26.39, 50.8816) (26.3295, 50.763) (26.2516, 50.656) knots 0 0 0 0 1 1 1 1
  line L367 (85.4087, 51.4947) -> (85.417, 51.9748)
  spline S1293 degree 3 poles (26.4924, 51.3965) (26.4925, 51.2644) (26.4717, 51.1331) (26.4309, 51.0074) knots 0 0 0 0 1 1 1 1
  spline S1294 degree 3 poles (25.9731, 52.4161) (26.08, 52.3382) (26.174, 52.2441) (26.2516, 52.137) knots 0 0 0 0 1 1 1 1
  spline S1295 degree 3 poles (23.9727, 51.3965) (23.9727, 51.7306) (24.1054, 52.0511) (24.3417, 52.2874) knots 0 0 0 0 1 1 1 1
  line L368 (82.7686, 46.9404) -> (82.8492, 51.5396)
  line L369 (73.0849, 54.9436) -> (73.0849, 53.9436)
  line L370 (78.0851, 46.7436) -> (76.7173, 46.7436)
  line L371 (85.7984, 46.8872) -> (82.7686, 46.9404)
  spline S1296 degree 3 poles (86.8184, 44.7003) (87.2048, 45.0867) (87.7288, 45.3038) (88.2752, 45.3038) knots 0 0 0 0 1 1 1 1
  line L372 (85.417, 51.9748) -> (85.9461, 52.4858)
  spline S1297 degree 3 poles (25.2326, 52.6564) (25.3647, 52.6564) (25.496, 52.6356) (25.6217, 52.5949) knots 0 0 0 0 1 1 1 1
  spline S1298 degree 3 poles (25.2326, 50.1366) (24.8984, 50.1366) (24.578, 50.2693) (24.3417, 50.5056) knots 0 0 0 0 1 1 1 1
  spline S1299 degree 3 poles (24.3417, 52.2874) (24.578, 52.5237) (24.8984, 52.6564) (25.2326, 52.6564) knots 0 0 0 0 1 1 1 1
  line L373 (73.5851, 53.4434) -> (78.0851, 53.4434)
  spline S1300 degree 3 poles (76.8351, 46.2438) (76.8352, 45.9095) (76.7025, 45.5888) (76.4661, 45.3524) knots 0 0 0 0 1 1 1 1
  line L374 (74.522, 46.7436) -> (72.069, 46.7436)
  spline S1301 degree 3 poles (74.3148, 46.2438) (74.3469, 46.4235) (74.4176, 46.5939) (74.522, 46.7436) knots 0 0 0 0 1 1 1 1
  spline S1302 degree 3 poles (88.808, 41.254) (88.6342, 41.2074) (88.4551, 41.1837) (88.2752, 41.1837) knots 0 0 0 0 1 1 1 1
  spline S1303 degree 3 poles (71.8592, 45.2134) (71.769, 45.0576) (71.6589, 44.9143) (71.5315, 44.7871) knots 0 0 0 0 1 1 1 1
  spline S1304 degree 3 poles (72.0648, 45.7105) (72.0183, 45.5366) (71.9492, 45.3694) (71.8592, 45.2134) knots 0 0 0 0 1 1 1 1
  spline S1305 degree 3 poles (24.3417, 50.5056) (24.1054, 50.7419) (23.9727, 51.0624) (23.9727, 51.3965) knots 0 0 0 0 1 1 1 1
  line L375 (78.0851, 47.6934) -> (78.0851, 46.7436)
  spline S1306 degree 3 poles (31.2446, 53.8656) (31.0708, 53.9122) (30.8917, 53.9358) (30.7118, 53.9359) knots 0 0 0 0 1 1 1 1
  line L376 (78.0851, 53.4434) -> (78.0851, 52.2936)
  spline S1307 degree 3 poles (30.7118, 53.9359) (30.1654, 53.9359) (29.6414, 53.7187) (29.2551, 53.3323) knots 0 0 0 0 1 1 1 1
  spline S1308 degree 3 poles (26.4309, 51.7861) (26.4718, 51.6603) (26.4925, 51.5288) (26.4924, 51.3965) knots 0 0 0 0 1 1 1 1
  line L377 (86.7327, 45.971) -> (85.7984, 46.8872)
  line L378 (89.809, 44.6) -> (89.81, 44.6672)
  spline S1309 degree 3 poles (88.2752, 45.3038) (88.4551, 45.3038) (88.6342, 45.2802) (88.808, 45.2336) knots 0 0 0 0 1 1 1 1
  spline S1310 degree 3 poles (73.2301, 53.5886) (73.3241, 53.4944) (73.4521, 53.4421) (73.5851, 53.4434) knots 0 0 0 0 1 1 1 1
  line L379 (72.5852, 55.4438) -> (73.0849, 54.9436)
  spline S1311 degree 3 poles (73.0849, 53.9436) (73.0836, 53.8106) (73.136, 53.6826) (73.2301, 53.5886) knots 0 0 0 0 1 1 1 1
  spline S1312 degree 3 poles (90.2647, 42.7102) (90.2182, 42.5364) (90.149, 42.3694) (90.0591, 42.2136) knots 0 0 0 0 1 1 1 1
  spline S1313 degree 3 poles (88.2752, 41.1837) (87.7289, 41.1836) (87.2048, 41.4005) (86.8184, 41.7868) knots 0 0 0 0 1 1 1 1
  line L380 (80.6602, 47.6934) -> (78.0851, 47.6934)
  spline S1314 degree 3 poles (90.0591, 42.2136) (89.9692, 42.0576) (89.8592, 41.9141) (89.732, 41.7868) knots 0 0 0 0 1 1 1 1
  line L381 (80.6602, 52.2936) -> (80.6602, 47.6934)
  spline S1315 degree 3 poles (75.5752, 44.9835) (75.2411, 44.9834) (74.9206, 45.1162) (74.6843, 45.3524) knots 0 0 0 0 1 1 1 1
  line L382 (82.8492, 51.5396) -> (85.4087, 51.4947)
  spline S1316 degree 3 poles (74.6843, 45.3524) (74.4477, 45.5888) (74.3148, 45.9094) (74.3148, 46.2438) knots 0 0 0 0 1 1 1 1
  spline S1317 degree 3 poles (72.069, 46.7436) (72.1114, 46.5803) (72.1336, 46.4125) (72.1351, 46.2438) knots 0 0 0 0 1 1 1 1
  spline S1318 degree 3 poles (86.2149, 43.2435) (86.2149, 43.7899) (86.432, 44.314) (86.8184, 44.7003) knots 0 0 0 0 1 1 1 1
  spline S1319 degree 3 poles (89.732, 44.7003) (89.7586, 44.6676) (89.7843, 44.6342) (89.809, 44.6) knots 0 0 0 0 1 1 1 1
  line L383 (25.2326, 52.6564) -> (25.2326, 52.6564)
  spline S1320 degree 3 poles (72.1351, 46.2438) (72.1351, 46.0638) (72.1115, 45.8845) (72.0648, 45.7105) knots 0 0 0 0 1 1 1 1
  spline S1321 degree 3 poles (76.4661, 45.3524) (76.2298, 45.1162) (75.9094, 44.9834) (75.5752, 44.9835) knots 0 0 0 0 1 1 1 1
  spline S1322 degree 3 poles (89.3051, 45.0274) (89.4611, 44.9375) (89.6046, 44.8275) (89.732, 44.7003) knots 0 0 0 0 1 1 1 1
  spline S1323 degree 3 poles (86.8184, 41.7868) (86.432, 42.1731) (86.2149, 42.6971) (86.2149, 43.2435) knots 0 0 0 0 1 1 1 1
  spline S1324 degree 3 poles (89.81, 44.6672) (89.7681, 45.0262) (89.5931, 45.3565) (89.3196, 45.5927) knots 0 0 0 0 1 1 1 1
  line L384 (67.585, 55.4438) -> (72.5852, 55.4438)
  spline S1325 degree 3 poles (89.3051, 41.4596) (89.1491, 41.3696) (88.982, 41.3005) (88.808, 41.254) knots 0 0 0 0 1 1 1 1
  spline S1326 degree 3 poles (25.9731, 50.3769) (25.8661, 50.2993) (25.7475, 50.2389) (25.6217, 50.1981) knots 0 0 0 0 1 1 1 1
  spline S1327 degree 3 poles (25.6217, 52.5949) (25.7475, 52.5541) (25.8661, 52.4937) (25.9731, 52.4161) knots 0 0 0 0 1 1 1 1
  spline S1328 degree 3 poles (26.2516, 52.137) (26.3294, 52.0302) (26.3899, 51.9118) (26.4309, 51.7861) knots 0 0 0 0 1 1 1 1
  spline S1329 degree 3 poles (106.918, 35.9406) (106.7442, 35.894) (106.5651, 35.8704) (106.3852, 35.8703) knots 0 0 0 0 1 1 1 1
  spline S1330 degree 3 poles (104.9284, 39.3869) (105.3148, 39.7733) (105.8388, 39.9905) (106.3852, 39.9905) knots 0 0 0 0 1 1 1 1
  spline S1331 degree 3 poles (106.918, 39.9202) (107.092, 39.8735) (107.2591, 39.8042) (107.4151, 39.714) knots 0 0 0 0 1 1 1 1
  spline S1332 degree 3 poles (30.7118, 49.8157) (30.8917, 49.8158) (31.0708, 49.8394) (31.2446, 49.886) knots 0 0 0 0 1 1 1 1
  spline S1333 degree 3 poles (31.2446, 49.886) (31.4186, 49.9325) (31.5857, 50.0017) (31.7417, 50.0917) knots 0 0 0 0 1 1 1 1
  line L385 (110.1441, 45.0036) -> (114.6415, 44.8465)
  spline S1334 degree 3 poles (113.0799, 38.1275) (113.1208, 38.0019) (113.1418, 37.8706) (113.1419, 37.7384) knots 0 0 0 0 1 1 1 1
  spline S1335 degree 3 poles (110.9906, 36.8475) (110.7544, 37.0838) (110.6216, 37.4043) (110.6216, 37.7384) knots 0 0 0 0 1 1 1 1
  spline S1336 degree 3 poles (107.842, 36.4734) (107.7146, 36.3462) (107.5711, 36.2362) (107.4151, 36.1463) knots 0 0 0 0 1 1 1 1
  spline S1337 degree 3 poles (104.3249, 37.9301) (104.3249, 38.4766) (104.542, 39.0006) (104.9284, 39.3869) knots 0 0 0 0 1 1 1 1
  spline S1338 degree 3 poles (29.2551, 50.4193) (29.6414, 50.0329) (30.1654, 49.8157) (30.7118, 49.8157) knots 0 0 0 0 1 1 1 1
  line L386 (114.6012, 43.6972) -> (117.1747, 43.6073)
  spline S1339 degree 3 poles (28.6515, 51.8761) (28.6515, 51.3296) (28.8686, 50.8056) (29.2551, 50.4193) knots 0 0 0 0 1 1 1 1
  line L387 (107.9422, 39.2562) -> (107.9448, 39.3264)
  spline S1340 degree 3 poles (107.842, 39.3869) (107.8771, 39.3447) (107.9106, 39.3011) (107.9422, 39.2562) knots 0 0 0 0 1 1 1 1
  line L388 (103.9724, 41.6167) -> (100.9442, 41.7227)
  line L389 (104.8902, 40.684) -> (103.9724, 41.6167)
  line L390 (103.6799, 46.71) -> (104.2179, 47.2117)
  spline S1341 degree 3 poles (31.7417, 50.0917) (31.8975, 50.1818) (32.0409, 50.2919) (32.1681, 50.4193) knots 0 0 0 0 1 1 1 1
  line L391 (44.8618, 45.1809) -> (44.8618, 45.1809)
  spline S1342 degree 3 poles (65.3159, 47.2629) (65.4228, 47.1852) (65.5168, 47.0912) (65.5944, 46.9844) knots 0 0 0 0 1 1 1 1
  spline S1343 degree 3 poles (65.7732, 46.633) (65.8142, 46.5073) (65.8351, 46.376) (65.8352, 46.2438) knots 0 0 0 0 1 1 1 1
  spline S1344 degree 3 poles (65.5944, 46.9844) (65.6721, 46.8773) (65.7324, 46.7588) (65.7732, 46.633) knots 0 0 0 0 1 1 1 1
  line L392 (104.2179, 47.2117) -> (109.2145, 47.0371)
  spline S1345 degree 3 poles (107.4704, 40.2607) (107.2009, 40.5018) (106.8507, 40.6329) (106.4891, 40.6282) knots 0 0 0 0 1 1 1 1
  spline S1346 degree 3 poles (65.4663, 45.3524) (65.2298, 45.116) (64.9092, 44.9833) (64.5748, 44.9835) knots 0 0 0 0 1 1 1 1
  spline S1347 degree 3 poles (63.6839, 47.1347) (63.9202, 47.371) (64.2407, 47.5037) (64.5748, 47.5037) knots 0 0 0 0 1 1 1 1
  spline S1348 degree 3 poles (107.4151, 36.1463) (107.2591, 36.0563) (107.092, 35.9871) (106.918, 35.9406) knots 0 0 0 0 1 1 1 1
  line L393 (64.5748, 47.5037) -> (64.5748, 47.5037)
  spline S1349 degree 3 poles (108.445, 37.9301) (108.445, 37.7501) (108.4214, 37.5708) (108.3747, 37.3968) knots 0 0 0 0 1 1 1 1
  spline S1350 degree 3 poles (106.3852, 39.9905) (106.5651, 39.9904) (106.7442, 39.9668) (106.918, 39.9202) knots 0 0 0 0 1 1 1 1
  line L394 (110.8438, 38.2748) -> (108.3882, 38.3606)
  spline S1351 degree 3 poles (112.7724, 36.8475) (112.5362, 36.6111) (112.2157, 36.4782) (111.8815, 36.478) knots 0 0 0 0 1 1 1 1
  spline S1352 degree 3 poles (64.5748, 47.5037) (64.7072, 47.5036) (64.8387, 47.4827) (64.9645, 47.4417) knots 0 0 0 0 1 1 1 1
  line L395 (109.2145, 47.0371) -> (109.6966, 46.5198)
  spline S1353 degree 3 poles (65.8352, 46.2438) (65.8354, 45.9095) (65.7026, 45.5888) (65.4663, 45.3524) knots 0 0 0 0 1 1 1 1
  spline S1354 degree 3 poles (113.0442, 38.1978) (113.0568, 38.1748) (113.0687, 38.1513) (113.0799, 38.1275) knots 0 0 0 0 1 1 1 1
  line L396 (117.1747, 43.6073) -> (117.014, 39.0102)
  spline S1355 degree 3 poles (106.3852, 35.8703) (105.8389, 35.8702) (105.3148, 36.0871) (104.9284, 36.4734) knots 0 0 0 0 1 1 1 1
  line L397 (106.4891, 40.6282) -> (104.8902, 40.684)
  spline S1356 degree 3 poles (64.9645, 47.4417) (65.0903, 47.4009) (65.2089, 47.3406) (65.3159, 47.2629) knots 0 0 0 0 1 1 1 1
  spline S1357 degree 3 poles (109.7943, 45.1607) (109.8851, 45.0634) (110.0112, 45.0068) (110.1441, 45.0036) knots 0 0 0 0 1 1 1 1
  spline S1358 degree 3 poles (107.4151, 39.714) (107.5711, 39.6241) (107.7146, 39.5141) (107.842, 39.3869) knots 0 0 0 0 1 1 1 1
  spline S1359 degree 3 poles (64.5748, 44.9835) (64.2407, 44.9834) (63.9202, 45.1162) (63.6839, 45.3524) knots 0 0 0 0 1 1 1 1
  line L398 (114.4075, 38.1503) -> (113.0442, 38.1978)
  spline S1360 degree 3 poles (32.1681, 50.4193) (32.2955, 50.5466) (32.4056, 50.6901) (32.4957, 50.8461) knots 0 0 0 0 1 1 1 1
  spline S1361 degree 3 poles (113.1419, 37.7384) (113.1418, 37.4042) (113.0089, 37.0837) (112.7724, 36.8475) knots 0 0 0 0 1 1 1 1
  spline S1362 degree 3 poles (110.6216, 37.7384) (110.6529, 37.9321) (110.729, 38.1158) (110.8438, 38.2748) knots 0 0 0 0 1 1 1 1
  spline S1363 degree 3 poles (29.2551, 53.3323) (28.8687, 52.9461) (28.6516, 52.4223) (28.6515, 51.8761) knots 0 0 0 0 1 1 1 1
  spline S1364 degree 3 poles (107.9448, 39.3264) (107.9093, 39.6863) (107.74, 40.0197) (107.4704, 40.2607) knots 0 0 0 0 1 1 1 1
  line L399 (101.1044, 46.3198) -> (103.6629, 46.2304)
  line L400 (103.6629, 46.2304) -> (103.6799, 46.71)
  line L401 (117.014, 39.0102) -> (114.441, 39.0996)
  spline S1365 degree 3 poles (108.3747, 37.3968) (108.3282, 37.223) (108.259, 37.0561) (108.1691, 36.9002) knots 0 0 0 0 1 1 1 1
  line L402 (100.9442, 41.7227) -> (101.1044, 46.3198)
  line L403 (114.441, 39.0996) -> (114.4075, 38.1503)
  spline S1366 degree 3 poles (109.662, 45.5204) (109.656, 45.3876) (109.7037, 45.258) (109.7943, 45.1607) knots 0 0 0 0 1 1 1 1
  line L404 (109.6966, 46.5198) -> (109.662, 45.5204)
  spline S1367 degree 3 poles (43.9709, 44.8119) (44.2072, 45.0481) (44.5277, 45.1809) (44.8618, 45.1809) knots 0 0 0 0 1 1 1 1
  spline S1368 degree 3 poles (111.8815, 36.478) (111.5473, 36.4782) (111.2268, 36.6111) (110.9906, 36.8475) knots 0 0 0 0 1 1 1 1
  spline S1369 degree 3 poles (108.1691, 36.9002) (108.0792, 36.7443) (107.9692, 36.6008) (107.842, 36.4734) knots 0 0 0 0 1 1 1 1
  spline S1370 degree 3 poles (104.9284, 36.4734) (104.542, 36.8597) (104.3249, 37.3837) (104.3249, 37.9301) knots 0 0 0 0 1 1 1 1
  line L405 (114.6415, 44.8465) -> (114.6012, 43.6972)
  spline S1371 degree 3 poles (108.3882, 38.3606) (108.4222, 38.2195) (108.4413, 38.0752) (108.445, 37.9301) knots 0 0 0 0 1 1 1 1
  spline S1372 degree 3 poles (30.4948, 46.8376) (30.1747, 46.8096) (29.8938, 46.613) (29.7579, 46.3219) knots 0 0 0 0 1 1 1 1
  spline S1373 degree 3 poles (51.3844, 42.425) (51.5404, 42.5149) (51.6839, 42.6248) (51.8113, 42.7521) knots 0 0 0 0 1 1 1 1
  spline S1374 degree 3 poles (43.602, 43.921) (43.602, 43.5868) (43.7347, 43.2664) (43.9709, 43.0301) knots 0 0 0 0 1 1 1 1
  spline S1375 degree 3 poles (46.1222, 43.921) (46.1222, 44.2551) (45.9895, 44.5756) (45.7533, 44.8119) knots 0 0 0 0 1 1 1 1
  line L406 (26.6361, 48.608) -> (25.3307, 48.4938)
  spline S1376 degree 3 poles (63.6839, 45.3524) (63.4476, 45.5888) (63.3148, 45.9095) (63.315, 46.2438) knots 0 0 0 0 1 1 1 1
  spline S1377 degree 3 poles (25.3307, 48.4938) (25.0107, 48.4655) (24.7301, 48.2688) (24.5944, 47.9776) knots 0 0 0 0 1 1 1 1
  spline S1378 degree 3 poles (45.7533, 43.0301) (45.9895, 43.2664) (46.1222, 43.5868) (46.1222, 43.921) knots 0 0 0 0 1 1 1 1
  line L407 (44.8618, 45.1809) -> (44.8618, 45.1809)
  spline S1379 degree 3 poles (46.1222, 43.921) (46.1222, 43.5868) (45.9895, 43.2664) (45.7533, 43.0301) knots 0 0 0 0 1 1 1 1
  spline S1380 degree 3 poles (52.3446, 43.6755) (52.3911, 43.8495) (52.4145, 44.0288) (52.4144, 44.2088) knots 0 0 0 0 1 1 1 1
  spline S1381 degree 3 poles (44.8618, 42.6611) (45.1962, 42.661) (45.5168, 42.7937) (45.7533, 43.0301) knots 0 0 0 0 1 1 1 1
  spline S1382 degree 3 poles (43.9709, 43.0301) (44.2072, 42.7938) (44.5277, 42.6611) (44.8618, 42.6611) knots 0 0 0 0 1 1 1 1
  spline S1383 degree 3 poles (27.5285, 47.3316) (27.6642, 47.6227) (27.6344, 47.964) (27.4505, 48.2272) knots 0 0 0 0 1 1 1 1
  spline S1384 degree 3 poles (32.0952, 53.3886) (31.9875, 53.4916) (31.869, 53.5825) (31.7417, 53.6599) knots 0 0 0 0 1 1 1 1
  spline S1385 degree 3 poles (45.7533, 44.8119) (45.5168, 45.0483) (45.1962, 45.181) (44.8618, 45.1809) knots 0 0 0 0 1 1 1 1
  spline S1386 degree 3 poles (27.4505, 48.2272) (27.6344, 47.964) (27.6642, 47.6227) (27.5285, 47.3316) knots 0 0 0 0 1 1 1 1
  line L408 (50.3545, 46.2686) -> (50.3545, 46.2686)
  spline S1387 degree 3 poles (31.7417, 53.6599) (31.5857, 53.7499) (31.4186, 53.8191) (31.2446, 53.8656) knots 0 0 0 0 1 1 1 1
  line L409 (31.8001, 46.9518) -> (31.8001, 46.9518)
  spline S1388 degree 3 poles (51.8113, 42.7521) (51.9385, 42.8794) (52.0485, 43.023) (52.1384, 43.1789) knots 0 0 0 0 1 1 1 1
  spline S1389 degree 3 poles (24.5944, 47.9776) (24.4585, 47.6864) (24.4883, 47.3449) (24.6724, 47.0815) knots 0 0 0 0 1 1 1 1
  line L410 (25.4878, 46.7012) -> (26.7927, 46.8149)
  spline S1390 degree 3 poles (24.5944, 47.9776) (24.7301, 48.2688) (25.0107, 48.4655) (25.3307, 48.4938) knots 0 0 0 0 1 1 1 1
  spline S1391 degree 3 poles (52.1384, 43.1789) (52.2285, 43.3347) (52.2979, 43.5017) (52.3446, 43.6755) knots 0 0 0 0 1 1 1 1
  spline S1392 degree 3 poles (44.8618, 45.1809) (45.1962, 45.181) (45.5168, 45.0483) (45.7533, 44.8119) knots 0 0 0 0 1 1 1 1
  spline S1393 degree 3 poles (45.7533, 43.0301) (45.5168, 42.7937) (45.1962, 42.661) (44.8618, 42.6611) knots 0 0 0 0 1 1 1 1
  spline S1394 degree 3 poles (27.5285, 47.3316) (27.393, 47.0404) (27.1126, 46.8435) (26.7927, 46.8149) knots 0 0 0 0 1 1 1 1
  line L411 (31.8001, 46.9518) -> (30.4948, 46.8376)